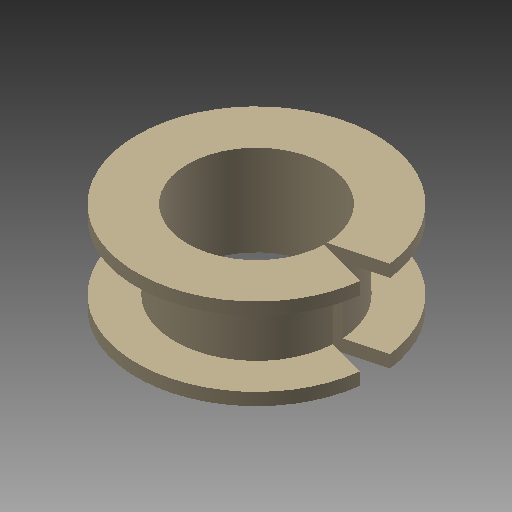
# Autodesk Inventor part: 311-04
Saved by Autodesk Inventor 2019 (Build 230136000, 136)
## iProperties
Company: Autodesk Inc.
Created: 2007-10-25
Part Number: 311-04
Document SubType Name: Modeling
Designer: Autodesk Inc.
Density: 8.47 g/cm^3
Mass: 2.09348 g
Surface Area: 7.3166 cm^2
Volume: 0.247164 cm^3
Material: Brass, Soft Yellow
Description: BUSHING 4 MM THICK
Appearance: Beige
Component Category: Fasteners
Author: Inventor
Autodesk Inventor part; units mm, degrees
ref_plane "YZ Plane" through (0, 0, 0) normal (1, 0, 0) x (0, 1, 0)
ref_plane "XZ Plane" through (0, 0, 0) normal (0, 1, 0) x (-1, 0, 0)
ref_plane "XY Plane" through (0, 0, 0) normal (0, 0, 1) x (1, 0, 0)
sketch "Sketch1" plane through (0, 0, 0) normal (0, 0, 1) x (1, 0, 0)
  line L0 (0, -3.85) -> (0, 3.85) projected
  line L1 (-1.45, 0) -> (8.7, 0) projected
  line L2 (4.18, -2.75) -> (4.18, 2.75)
  line L3 (4.18, 2.75) -> (7.25, 2.75)
  line L4 (7.25, 2.75) -> (7.25, 2)
  line L5 (7.25, 2) -> (4.945, 2)
  line L6 (4.945, 2) -> (4.945, -2)
  line L7 (4.945, -2) -> (7.25, -2)
  line L8 (7.25, -2) -> (7.25, -2.75)
  line L9 (7.25, -2.75) -> (4.18, -2.75)
  point P0 (0, 0)
  point P1 (4.945, 0)
  dimension "d0" = 8.36
  dimension "d1" = 9.89
  dimension "d2" = 14.5
  dimension "d3" = 0.75
  dimension "d4" = 4
  dimension "d5" = 0.75
  constraints: 16 end point, 6 parallel, 2 perpendicular, 1 collinear, 1 midpoint, 1 point on line
  measures "d0" diameter of L2 L0
  measures "d1" diameter of L6 L0
  measures "d2" diameter of L4 L0
  measures "d3" distance between parallel lines of L7 L9
  measures "d4" distance between parallel lines of L5 L7
  measures "d5" distance between parallel lines of L3 L5
revolve "Revolution1" add sketch "Sketch1" angle 360 about axis through (0, -10, 0) along (0, 1, 0)
sketch "Sketch3" plane through (0, 2.75, 0) normal (0, 1, 0) x (1, 0, 0)
  circle A0 centre (0, 0) radius 7.25 projected
  circle A1 centre (0, 0) radius 4.18 projected
  line L0 (-10.15, 0) -> (10.15, 0) projected
  line L1 (0, 10.15) -> (0, -10.15) projected
  line L2 (4.1788, 0.1015) -> (7.1928, 0.9091)
  line L3 (4.1788, -0.1015) -> (7.1928, -0.9091)
  arc A2 (4.1788, -0.1015) -> (4.1788, 0.1015) centre (0, 0) ccw
  arc A3 (7.1928, -0.9091) -> (7.1928, 0.9091) centre (0, 0) ccw
  dimension "d15" = 15
  dimension "d16" = 30
  dimension "d17" = 3.014
  dimension "d18" = 3.014
  constraints: 8 point on circle, 4 end point, 2 centre point, 2 coincident
  measures "d15" angle of L0 L3
  measures "d16" angle of L2 L3
  measures "d17" horizontal distance of L2.start L2.end
  measures "d18" horizontal distance of L3.start L3.end
extrude "Extrusion2" cut sketch "Sketch3" against normal through all contours L0 A1 L2 A0 | A0 L3 A1 L0
equation "\"d3\" = d5"
body "Solid1"
